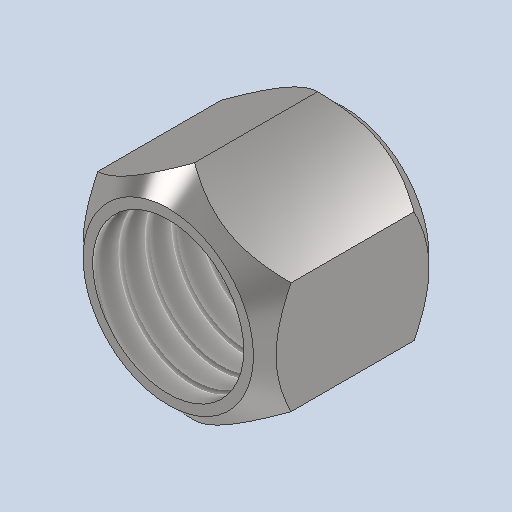
# Autodesk Inventor part: L3 Part 7
Saved by Autodesk Inventor 2024 (Build 280153000, 153)
## iProperties
Created: 2023-05-29
Part Number: L3 Part 7
Material: Stainless Steel
Document SubType Name: Modeling
Designer: vilas
Density: 8 g/cm^3
Appearance: Semi-Polished
Author: vilas
Autodesk Inventor part; units mm, degrees
ref_plane "YZ Plane" through (0, 0, 0) normal (1, 0, 0) x (0, 1, 0)
ref_plane "XZ Plane" through (0, 0, 0) normal (0, 1, 0) x (-1, 0, 0)
ref_plane "XY Plane" through (0, 0, 0) normal (0, 0, 1) x (1, 0, 0)
sketch "Sketch1" plane through (0, 0, 0) normal (0, 0, 1) x (1, 0, 0)
  circle A0 centre (0, 0) radius 2.15
  circle A1 centre (0, 0) radius 2.75
  line L0 (0, 3.1754) -> (2.75, 1.5877)
  line L1 (2.75, 1.5877) -> (2.75, -1.5877)
  line L2 (2.75, -1.5877) -> (0, -3.1754)
  line L3 (0, -3.1754) -> (-2.75, -1.5877)
  line L4 (-2.75, -1.5877) -> (-2.75, 1.5877)
  line L5 (-2.75, 1.5877) -> (0, 3.1754)
  dimension "d0" = 4.3
  dimension "d1" = 5.5
  constraints: 12 end point, 3 coincident, 2 centre point, 1 tangent, 1 vertical, 13 other
  measures "d0" diameter of A0
  measures "d1" diameter of A1
extrude "Extrusion1" add sketch "Sketch1" along normal mid plane 5
sketch "Sketch2" plane through (0, 0, 0) normal (1, 0, 0) x (0, 1, 0)
  line L0 (3.1754, 2.5) -> (1.5877, 2.5) projected
  line L1 (3.1754, 2.5) -> (3.1754, 1.75)
  line L2 (3.1754, 2.5) -> (2.4254, 2.5)
  line L3 (2.4254, 2.5) -> (3.1754, 1.75)
  line L4 (1.5877, 2.5) -> (-1.5877, 2.5) projected
  line L5 (0, 2.5) -> (0, -2.5) construction
  line L6 (2.15, -2.5) -> (-2.15, -2.5) projected
  line L7 (1.5877, -2.5) -> (3.1754, -2.5) projected
  line L8 (3.1754, -2.5) -> (3.1754, -1.75)
  line L9 (3.1754, -2.5) -> (2.4254, -2.5)
  line L10 (2.4254, -2.5) -> (3.1754, -1.75)
  point P0 (0, 0)
  dimension "d4" = 0.75
  dimension "d5" = 0.75
  dimension "d6" = 0.75
  dimension "d7" = 0.75
  constraints: 14 end point, 2 midpoint, 2 point on line, 2 vertical
  measures "d4" distance of L0.start L1.end
  measures "d5" distance of L0.start L2.end
  measures "d6" distance of L7.end L8.end
  measures "d7" distance of L7.end L9.end
revolve "Revolution1" cut sketch "Sketch2" angle 360 about axis through (0, 0, 2.5) along (0, 0, -1)
thread "Thread3" size "M4.5x0.75" class "6H" standard "ANSI Metric M Profile" length 5
body "Solid1"
